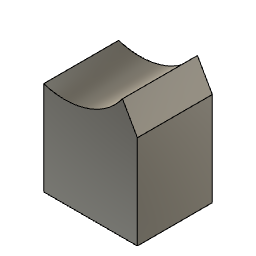
base Copy v1 (Autodesk Fusion 360 archive; units mm, degrees)
design "switch"
Autodesk Fusion 360 part; units mm, degrees
sketch "Sketch1" plane through (0, 0, 0) normal (0, 1, 0) x (1, 0, 0)
  line L0 (-5, -5) -> (-5, 5)
  line L1 (-5, 5) -> (5, 5)
  line L2 (5, 5) -> (5, -5)
  line L3 (5, -5) -> (-5, 5) construction
  line L4 (-5, -5) -> (5, 5) construction
  line L5 (5, -5) -> (3.4093, -7.8067)
  arc A0 (3.4093, -7.8067) -> (-5, -5) centre (-2.7358, -12.2173) ccw
  dimension "d1" = 10
  dimension "d2" = 10
  dimension "d4" = 3.2261
  constraint parallel L0 L2
  constraint coincident L3 origin
  constraint coincident L4 origin
  measures "d1" distance of L0.end L1.end
  measures "d2" distance of L0.start L0.end
  measures "d4" distance of L2.end L5.end
extrude "Extrude1" add sketch "Sketch1" along normal blind 8

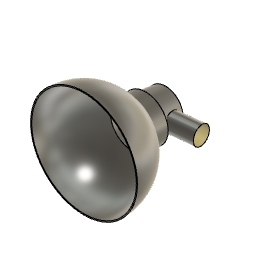
design "holder"
Autodesk Fusion 360 part; units mm, degrees
sketch "Sketch2" plane through (0, 0, 0) normal (0, 0, 1) x (1, 0, 0)
  line L0 (100, 0) -> (0, 0)
  arc A0 (100, 0) -> (42.0729, 90.7186) centre (0, 0) ccw
  line L1 (42.0729, 90.7186) -> (42.0729, 115.3624)
  line L2 (0, 152.3329) -> (0, 0)
  line L3 (32.8711, 152.4721) -> (0, 152.3329)
  line L4 (32.8711, 152.4721) -> (36.9604, 115.5405)
  line L5 (36.9604, 115.5405) -> (0, 115.5405)
  line L6 (42.0729, 115.3624) -> (36.9604, 115.5405)
  line L7 (42.0729, 90.7186) -> (0, 90.7186)
  dimension "d3" = 200
  constraint coincident L0.end A0.centre
  constraint horizontal L0
  constraint perpendicular L0 L2
  constraint symmetric L3.end L2 L2.start
  constraint perpendicular L2 L5
  constraint coincident L2 L7.end
  constraint perpendicular L2 L7
  measures "d3" diameter of A0
revolve "Revolve1" add sketch "Sketch2" angle 360 about axis through (0, 152.3329, 0) along (0, -1, 0) makes body 1
shell "Shell1" thickness 2 removed faces 1 at (-27.1036, 0, -4.9681) on bodies 1
ref_plane "WorkPlane1" through (34.9157, 134.0063, 0) normal (0.993926, 0.110055, 0) x (0, 0, -1)
ref_plane "WorkPlane2" through (30.94, 133.5661, 0) normal (0.993926, 0.110055, 0) x (0, 0, -1)
sketch "Sketch3" plane through (30.94, 133.5661, 0) normal (0.993926, 0.110055, 0) x (0, 0, -1)
  circle A0 centre (0, 0) radius 17
  dimension "d10" = 34
  constraint coincident A0.centre origin
  measures "d10" diameter of A0
surface "Extrude1" add extruded along (0.993926, 0.110055, 0) between 0 and 50 path "Sketch3" along A0 separate body makes body 2

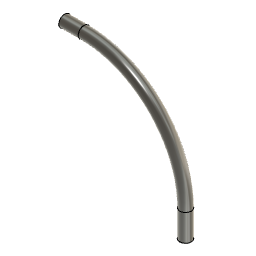
design "pipe"
Autodesk Fusion 360 part; units mm, degrees
sketch "Sketch1" plane through (0, 0, 0) normal (0, 0, 1) x (1, 0, 0)
  circle A0 centre (0, 0) radius 15
  circle A1 centre (0, 0) radius 13
  dimension "d1" = 30
  dimension "d2" = 26
  constraint coincident A0.centre A1.centre
  measures "d1" diameter of A0
  measures "d2" diameter of A1
sketch "Sketch2" plane through (0, 0, 0) normal (0, 1, 0) x (1, 0, 0)
  line L0 (0, 0) -> (0, -68.58)
  arc A0 (-260.84, -329.42) -> (0, -68.58) centre (-260.84, -68.58) ccw
  line L1 (-260.84, -329.42) -> (-310.84, -329.42)
  dimension "d3" = 68.58
  dimension "d4" = 260.84
  dimension "d5" = 50
  constraint coincident L0.start origin
  constraint vertical L0
  constraint tangent L0 A0
  constraint horizontal L1
  constraint vertical A0.start A0.centre
  measures "d3" distance of L0.start L0.end
  measures "d4" radius of A0
  measures "d5" distance of A0.start L1.end
sweep "Sweep1" add profiles "Sketch1" path "Sketch2" along L1 A0 L0 section 1
